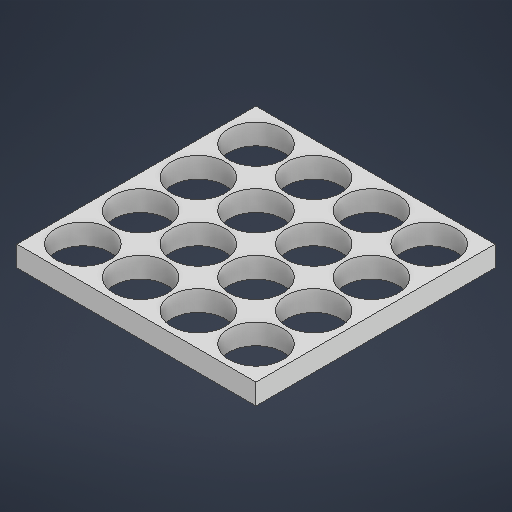
# Autodesk Inventor part: battery_pack_16s
Saved by Autodesk Inventor 2026.1 (Build 301233000, 233)
## iProperties
Created: 2026-03-08
Part Number: battery_pack_16s
Material: Generic
Document SubType Name: Modeling
Designer: aaron
Density: 1 g/cm^3
Appearance: Default
Author: aaron
Autodesk Inventor part; units mm, degrees
ref_plane "YZ Plane" through (0, 0, 0) normal (1, 0, 0) x (0, 1, 0)
ref_plane "XZ Plane" through (0, 0, 0) normal (0, 1, 0) x (-1, 0, 0)
ref_plane "XY Plane" through (0, 0, 0) normal (0, 0, 1) x (1, 0, 0)
sketch "Sketch1" plane through (0, 0, 0) normal (0, 1, 0) x (-1, 0, 0)
  circle A0 centre (10.7499, 10.3753) radius 13.1
  line L0 (10.7499, 10.3753) -> (10.7499, 16.4412)
  line L1 (10.7499, 10.3753) -> (17.5689, 10.3753)
  circle A1 centre (10.7499, 38.3753) radius 13.1
  circle A2 centre (10.7499, 66.3753) radius 13.1
  circle A3 centre (10.7499, 94.3753) radius 13.1
  circle A4 centre (38.7499, 10.3753) radius 13.1
  circle A5 centre (38.7499, 38.3753) radius 13.1
  circle A6 centre (38.7499, 66.3753) radius 13.1
  circle A7 centre (38.7499, 94.3753) radius 13.1
  circle A8 centre (66.7499, 10.3753) radius 13.1
  circle A9 centre (66.7499, 38.3753) radius 13.1
  circle A10 centre (66.7499, 66.3753) radius 13.1
  circle A11 centre (66.7499, 94.3753) radius 13.1
  circle A12 centre (94.7499, 10.3753) radius 13.1
  circle A13 centre (94.7499, 38.3753) radius 13.1
  circle A14 centre (94.7499, 66.3753) radius 13.1
  circle A15 centre (94.7499, 94.3753) radius 13.1
  line L2 (110.7499, 110.3753) -> (-5.2501, 110.3753)
  line L3 (-5.2501, 110.3753) -> (-5.2501, -5.6247)
  line L4 (-5.2501, -5.6247) -> (110.7499, -5.6247)
  line L5 (110.7499, -5.6247) -> (110.7499, 110.3753)
  point P0 (0, 0)
  dimension "d0" = 26.2
  dimension "d3" = 28
  dimension "d6" = 28
  dimension "d9" = 16
  dimension "d10" = 16
  dimension "d11" = 16
  dimension "d12" = 16
  constraints: 16 centre point, 12 end point, 3 horizontal, 2 parallel, 2 vertical, 1 perpendicular, 30 other
  measures "d0" diameter of A0
  measures "d3" distance of L0.start A1.centre
  measures "d6" distance of L0.start A4.centre
  measures "d9" distance from line of L5 A15.centre
  measures "d10" distance from line of L3 A3.centre
  measures "d11" distance from line of L2 A15.centre
  measures "d12" distance from line of L4 A12.centre
extrude "Extrusion1" add sketch "Sketch1" along normal blind 10
equation "\"d10\" = d9"
equation "\"d11\" = d9"
equation "\"d12\" = d9"
body "Solid1"
